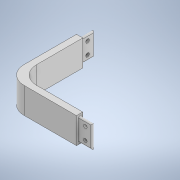
# Autodesk Inventor part: Joint
Saved by Autodesk Inventor 2021 (Build 250183000, 183)
## iProperties
Created: 2024-01-09
Part Number: Joint
Material: Generic
Document SubType Name: Modeling
Designer: brybr
Density: 1 g/cm^3
Appearance: Default
Author: brybr
Autodesk Inventor part; units mm, degrees
sketch "Sketch1" plane through (0, 0, 0) normal (0, 1, 0) x (-1, 0, 0)
  line L0 (0, 0) -> (90, 0) construction
  line L1 (90, 0) -> (90, -90) construction
  line L2 (90, -90) -> (90, 0)
  line L3 (0, 0) -> (90, 0)
  dimension "d2" = 90
  dimension "d3" = 90
  dimension "d4" = 90
  constraints: 8 end point, 2 perpendicular, 1 collinear, 1 horizontal
  measures "d2" distance of L0.start L0.end
  measures "d3" distance of L0.end L1.end
  measures "d4" angle of L0 L1
sketch "Sketch2" plane through (0, 0, 0) normal (1, 0, 0) x (0, 1, 0)
  line L0 (12.4, 1.25) -> (-12.4, 1.25)
  line L1 (-12.4, 1.25) -> (-12.4, -1.25)
  line L2 (-12.4, -1.25) -> (12.4, -1.25)
  line L3 (12.4, -1.25) -> (12.4, 1.25)
  line L4 (12.4, 1.25) -> (-12.4, -1.25) construction
  line L5 (-12.4, 1.25) -> (12.4, -1.25) construction
  line L6 (12.4, 1.25) -> (37.2, 1.25) construction
  point P0 (0, 0)
  dimension "d5" = 24.8
  dimension "d6" = 180
  dimension "d7" = 2.5
  constraints: 14 end point, 2 horizontal, 2 midpoint, 2 parallel, 1 collinear, 1 perpendicular
  measures "d5" distance of L0.start L0.end
  measures "d6" angle of L0 L6
  measures "d7" distance of L1.end L0.end
sweep "Sweep1" add profiles "Sketch2" path "Sketch1" path curves L3 L2
sketch "Sketch3" plane through (0, 0, 0) normal (0, 1, 0) x (-1, 0, 0)
  line L0 (40, 0) -> (40, 0) construction
  line L1 (0, -1.25) -> (88.75, -1.25) construction
  line L2 (40, 0) -> (40, 0) construction
  line L3 (40, 0) -> (40, 0) construction
  line L4 (40, 0) -> (40, 0) construction
  line L5 (88.75, -1.25) -> (88.75, -90) construction
  line L6 (88.75, -48.75) -> (41.25, -1.25)
  point P0 (0, 0)
  point P1 (0.5, -1)
  point P2 (39, -39.5)
  dimension "d14" = 0
  dimension "d15" = 180
  dimension "d16" = 45
  constraints: 10 end point, 2 horizontal, 2 point on line, 1 collinear, 1 vertical, 4 other
  measures "d14" distance of L0.start L0.end
  measures "d15" angle of L2 L0
  measures "d16" angle of L3 L0
feature "Rib1" [suppressed]
pattern_linear "Rectangular Pattern1" [suppressed]
pattern_linear "Rectangular Pattern2" [suppressed]
ref_plane "Work Plane2" through (-39, -12.4, -39.5) normal (1, 0, 0) x (0, 0, -1)
ref_plane "Work Plane1" through (-91.25, -6.2, 1.25) normal (-0.7071068, 0, -0.7071068) x (0, 1, 0)
sketch "Sketch5" plane through (-88.75, -12.4, -90) normal (1, 0, 0) x (0, 0, -1)
  line L0 (-88.75, 0) -> (0, 0) construction
  line L1 (0, 0) -> (-7.5, 0) construction
  line L2 (0, 0) -> (7.5, 0) construction
  circle A0 centre (-7.5, 5.65) radius 2
  circle A1 centre (-7.5, 19.15) radius 2
  line L3 (-91.25, 0) -> (0, 0) construction
  line L4 (-7.5, 0) -> (-7.5, 5.65) construction
  line L5 (-7.5, 19.15) -> (-7.5, 24.8) construction
  line L6 (-91.25, 24.8) -> (0, 24.8) construction
  line L7 (-7.5, 19.15) -> (-7.5, 5.65) construction
  point P0 (-90, 12.4)
  dimension "d43" = 7.5
  dimension "d44" = 180
  dimension "d47" = 4
  dimension "d49" = 4
  dimension "d63" = 13.5
  constraints: 10 end point, 3 collinear, 2 centre point, 2 horizontal, 2 vertical, 1 point on line
  measures "d43" distance of L0.end L1.end
  measures "d44" angle of L1 L2
  measures "d47" diameter of A0
  measures "d49" diameter of A1
  measures "d63" distance of L5.start L4.end
extrude "Extrusion2" cut sketch "Sketch5" against normal up to next
mirror "Mirror3" about plane through (-91.25, -6.2, 1.25) normal (-0.7071068, 0, -0.7071068) of "Extrusion2"
sketch "Sketch6" plane through (0, 0, 0) normal (0, 1, 0) x (-1, 0, 0)
  line L0 (15, 0) -> (90, 0)
  line L1 (15, 0) -> (90, 0) construction
  line L2 (90, 0) -> (90, -75)
  point P0 (0, 0)
  dimension "d52" = 75
  dimension "d53" = 0
  dimension "d54" = 75
  dimension "d55" = 90
  constraints: 6 end point, 2 horizontal, 1 collinear, 1 perpendicular
  measures "d52" distance of L0.start L0.end
  measures "d53" distance between parallel lines of L0 L1
  measures "d54" distance of L0.end L2.end
  measures "d55" angle of L0 L2
ref_plane "Work Plane3" through (-15, -12.4, -1.25) normal (1, 0, 0) x (0, 0, -1)
sketch "Sketch7" plane through (-15, -12.4, -1.25) normal (1, 0, 0) x (0, 0, -1)
  line L0 (-4.75, 26.9) -> (-4.75, -2.1)
  line L1 (-4.75, -2.1) -> (2.25, -2.1)
  line L2 (2.25, -2.1) -> (2.25, 26.9)
  line L3 (2.25, 26.9) -> (-4.75, 26.9)
  line L4 (-4.75, 26.9) -> (2.25, -2.1) construction
  line L5 (-4.75, -2.1) -> (2.25, 26.9) construction
  line L6 (-4.75, 26.9) -> (24.25, 26.9) construction
  point P0 (-1.25, 12.4)
  dimension "d57" = 29
  dimension "d58" = 90
  dimension "d59" = 7
  constraints: 14 end point, 2 midpoint, 2 parallel, 2 perpendicular, 1 horizontal, 1 vertical
  measures "d57" distance of L0.start L0.end
  measures "d58" angle of L0 L6
  measures "d59" distance of L1.end L0.end
sweep "Sweep2" add profiles "Sketch7" path "Sketch6"
fillet "Fillet3" radius 1.25 12 edges at (0, 0, -1.25) (0, 0, 1.25) (-88.75, 0, -90) (-91.25, 0, -90) (-7.5, 12.4, 1.25) (-7.5, 12.4, -1.25) (-91.25, 12.4, -82.5) (-88.75, 12.4, -82.5) (-91.25, -12.4, -82.5) (-88.75, -12.4, -82.5) (-7.5, -12.4, 1.25) (-7.5, -12.4, -1.25)
fillet "Fillet4" radius 20 2 edges at (-86.5, 0, -3.5) (-93.5, 0, 3.5)
body "Solid1"
